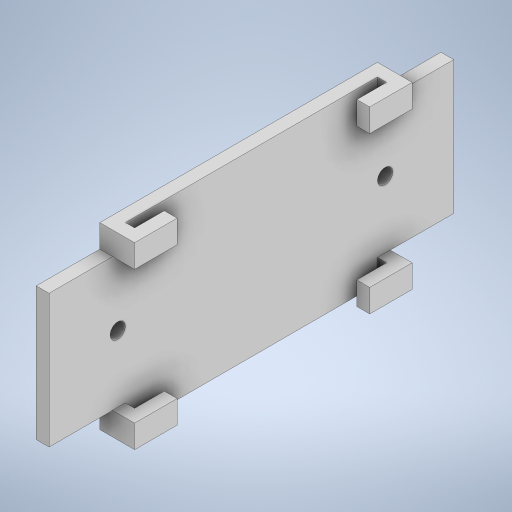
# Autodesk Inventor part: cam_holder2_conv
Saved by Autodesk Inventor 2024.3 (Build 283343000, 343)
## iProperties
Created: 2024-12-19
Part Number: cam_holder2_conv
Material: Generic
Document SubType Name: Modeling
Designer: User
Density: 1 g/cm^3
Appearance: Default
Author: User
Autodesk Inventor part; units mm, degrees
ref_plane "YZ Plane" through (0, 0, 0) normal (1, 0, 0) x (0, 1, 0)
ref_plane "XZ Plane" through (0, 0, 0) normal (0, 1, 0) x (-1, 0, 0)
ref_plane "XY Plane" through (0, 0, 0) normal (0, 0, 1) x (1, 0, 0)
sketch "Sketch1" plane through (0, 0, 0) normal (0, 1, 0) x (-1, 0, 0)
  line L0 (0, 27.1) -> (0, -27.1)
  line L1 (0, 27.1) -> (-6.8, 27.1)
  line L2 (-6.8, 27.1) -> (-6.8, 18.8)
  line L3 (-6.8, 18.8) -> (-4.3, 18.8)
  line L4 (-4.3, 18.8) -> (-4.3, 24.6)
  line L5 (-4.3, 24.6) -> (-2.5, 24.6)
  line L6 (-2.5, 24.6) -> (-2.5, 0)
  line L7 (0, -27.1) -> (-6.8, -27.1)
  line L8 (-6.8, -27.1) -> (-6.8, -18.8)
  line L9 (-6.8, -18.8) -> (-4.3, -18.8)
  line L10 (-4.3, -18.8) -> (-4.3, -24.6)
  line L11 (-4.3, -24.6) -> (-2.5, -24.6)
  line L12 (-2.5, -24.6) -> (-2.5, 0)
  point P0 (0, 0)
  dimension "d0" = 54.2
  dimension "d1" = 6.8
  dimension "d2" = 8.3
  dimension "d3" = 2.5
  dimension "d4" = 5.8
  dimension "d5" = 1.8
  dimension "d6" = 8.3
  dimension "d7" = 5.8
  constraints: 26 end point, 5 perpendicular, 4 horizontal, 3 vertical, 1 parallel
  measures "d0" distance of L0.start L0.end
  measures "d1" distance of L0.start L1.end
  measures "d2" distance of L1.end L2.end
  measures "d3" distance of L2.end L3.end
  measures "d4" distance of L3.end L4.end
  measures "d5" distance of L4.end L5.end
  measures "d6" distance of L7.end L8.end
  measures "d7" distance of L9.end L10.end
extrude "Extrusion1" add sketch "Sketch1" along normal blind 4.5
sketch "Sketch2" plane through (0, 4.5, 0) normal (0, 1, 0) x (1, 0, 0)
  line L0 (2.5, -24.6) -> (2.5, 24.6) projected
  line L1 (2.5, 0) -> (2.5, 39.5)
  line L2 (2.5, 39.5) -> (0, 39.5)
  line L3 (0, 39.5) -> (0, 0)
  line L4 (0, 0) -> (0, -39.5)
  line L5 (0, 27.1) -> (0, -27.1) projected
  line L6 (0, -39.5) -> (2.5, -39.5)
  line L7 (2.5, -39.5) -> (2.5, 0)
  dimension "d10" = 39.5
  dimension "d11" = 39.5
  constraints: 12 end point, 3 collinear, 2 perpendicular, 1 midpoint
  measures "d10" distance of L1.start L1.end
  measures "d11" distance of L3.end L4.end
extrude "Extrusion2" add sketch "Sketch2" along normal blind 26
sketch "Sketch3" plane through (0, 30.5, 0) normal (0, 1, 0) x (1, 0, 0)
  line L0 (2.5, -24.6) -> (2.5, 24.6) projected
  line L1 (2.5, 0) -> (2.5, 24.6558)
  line L2 (0, 27.1) -> (0, -27.1) projected
  line L3 (4.3, -24.6) -> (2.5, -24.6) projected
  line L4 (6.8, -18.8) -> (4.3, -18.8) projected
  line L5 (4.3, -24.6) -> (4.3, -18.8)
  line L6 (4.3, -18.8) -> (6.8, -18.8)
  line L7 (6.8, -18.8) -> (6.8, -27.1)
  line L8 (6.8, -27.1) -> (2.5, -27.1)
  line L9 (2.5, 0) -> (2.5, 24.6558)
  line L10 (2.5, 24.6) -> (4.3, 24.6) projected
  line L11 (4.3, 18.8) -> (6.8, 18.8) projected
  line L12 (4.3, 24.6) -> (4.3, 18.8)
  line L13 (4.3, 18.8) -> (6.8, 18.8)
  line L14 (6.8, 18.8) -> (6.8, 27.1)
  line L15 (6.8, 27.1) -> (0, 27.1)
  line L16 (0, 27.1) -> (0, -27.1)
  line L17 (6.8, -27.1) -> (0, -27.1)
  line L18 (4.3, -24.6) -> (2.5, -24.6)
  point P0 (0, 0)
  constraints: 26 end point, 6 perpendicular, 2 collinear, 2 parallel, 2 vertical, 1 midpoint
extrude "Extrusion3" add sketch "Sketch3" along normal blind 4.5
sketch "Sketch4" plane through (2.5, 0, 24.6) normal (1, 0, 0) x (0, 0, -1)
  line L0 (64.1, 4.5) -> (64.1, 30.5) projected
  line L1 (64.1, 17.5) -> (50.7, 17.5)
  circle A0 centre (50.7, 17.5) radius 1.5
  line L2 (-14.9, 4.5) -> (-14.9, 30.5) projected
  line L3 (-14.9, 17.5) -> (-1.5, 17.5)
  circle A1 centre (-1.5, 17.5) radius 1.5
  point P0 (24.6, 0)
  dimension "d16" = 13.4
  dimension "d17" = 3
  dimension "d18" = 13.4
  dimension "d19" = 3
  constraints: 4 end point, 2 centre point, 2 coincident, 2 horizontal, 2 midpoint
  measures "d16" distance of L1.start L1.end
  measures "d17" diameter of A0
  measures "d18" distance of L3.start L3.end
  measures "d19" diameter of A1
extrude "Extrusion4" cut sketch "Sketch4" against normal blind 4.5
body "Solid1"
